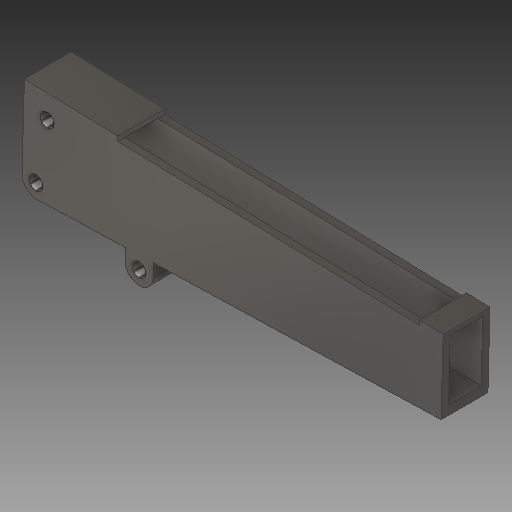
# Autodesk Inventor part: DipperParent
Saved by Autodesk Inventor 2019 (Build 230136000, 136)
## iProperties
Created: 2018-12-27
Part Number: DipperParent
Material: 钢，高强度，低合金
Document SubType Name: Modeling
Designer: JianQiao Hu
Density: 7.85 g/cm^3
Appearance: 钢 - 抛光
Author: JianQiao Hu
Autodesk Inventor part; units mm, degrees
ref_plane "YZ Plane" through (0, 0, 0) normal (1, 0, 0) x (0, 1, 0)
ref_plane "XZ Plane" through (0, 0, 0) normal (0, 1, 0) x (-1, 0, 0)
ref_plane "XY Plane" through (0, 0, 0) normal (0, 0, 1) x (1, 0, 0)
sketch "草图1" plane through (0, 0, 0) normal (0, 0, 1) x (1, 0, 0)
  line L0 (598.9577, 75) -> (600, -74.9964)
  line L1 (-601.0423, 75.1267) -> (600, -74.9964) construction
  line L2 (598.9577, 75) -> (-593.8092, -74.3553) construction
  line L3 (-300, 0) -> (-300, 100)
  line L4 (-300, -100) -> (600, -74.9964)
  line L5 (-300, 100) -> (598.9577, 75)
  line L6 (-300, 0) -> (-300, -100)
  line L7 (599.4789, 0) -> (-300, 0)
  line L8 (0, 0) -> (0, -189.9048)
  dimension "d0" = 150
  dimension "d31" = 75
  dimension "d32" = 0
  dimension "d33" = 100
  dimension "d34" = 100
  dimension "d35" = 100
  dimension "d51" = 300
  constraints: 18 end point, 5 point on line, 3 vertical, 1 perpendicular
  measures "d0" distance of L0.start L0.end
  measures "d31" distance from line of L0.start L7
  measures "d32" distance from line of L8.start L7
  measures "d33" distance from line of L3.end L7
  measures "d34" distance of L3.start L3.end
  measures "d35" distance of L3.start L4.start
  measures "d51" distance between parallel lines of L8 L6
extrude "拉伸1" add sketch "草图1" along normal mid plane 100
sketch "草图2" plane through (0, 0, 0) normal (0, 0, 1) x (1, 0, 0)
  circle A0 centre (-50, -120) radius 15
  line L0 (0, 0) -> (0, -405.8359)
  line L1 (0, 0) -> (-641.787, 0)
  line L2 (-80, -120) -> (-80, -93.888)
  line L3 (-300, -100) -> (600, -74.9964) projected
  line L4 (-20, -92.2211) -> (-20, -120)
  arc A1 (-80, -120) -> (-20, -120) centre (-50, -120) ccw
  dimension "d8" = 30
  dimension "d9" = 120
  dimension "d10" = 50
  dimension "d28" = 30
  constraints: 8 end point, 2 centre point, 2 point on circle, 2 point on line, 2 vertical, 1 coincident, 1 horizontal, 1 tangent
  measures "d8" diameter of A0
  measures "d9" distance from line of L1 A0.centre
  measures "d10" distance from line of L0 A0.centre
  measures "d28" radius of A1
extrude "拉伸2" add sketch "草图2" along normal mid plane 100
fillet "圆角1" radius 30 1 edges at (-300, -100, 0)
sketch "草图4" plane through (0, 0, 50) normal (0, 0, 1) x (1, 0, 0)
  arc A0 (-300, -69.155) -> (-269.1669, -99.1434) centre (-270, -69.155) ccw projected
  circle A1 centre (-270, -69.155) radius 15
  point P0 (0, 0)
  dimension "d15" = 30
  constraints: 1 centre point, 1 coincident
  measures "d15" diameter of A1
extrude "拉伸3" cut sketch "草图4" against normal blind 100
sketch "草图5" plane through (0, 0, 50) normal (0, 0, 1) x (1, 0, 0)
  arc A0 (-300, -69.155) -> (-269.1669, -99.1434) centre (-270, -69.155) ccw projected
  line L0 (-300, -69.155) -> (-300, 100)
  line L1 (598.9577, 75) -> (-300, 100) projected
  line L2 (-300, 100) -> (-300, -69.155) projected
  line L3 (-300, 100) -> (-300, 100)
  line L4 (-300, -69.155) -> (-295.2994, 99.8693)
  line L5 (-295.2994, 99.8693) -> (-300, 100)
  line L6 (598.9577, 75) -> (594.7823, -75.1413)
  line L7 (600, -74.9964) -> (-269.1669, -99.1434) projected
  line L8 (598.9577, 75) -> (600, -74.9964) projected
  line L9 (600, -74.9964) -> (598.9577, 75)
  point P0 (0, 0)
  point P1 (-603.2218, 0)
  point P2 (599.4789, 0)
  dimension "d20" = 90
  constraints: 12 end point, 3 point on line, 1 collinear, 1 horizontal, 1 parallel, 1 other
  measures "d20" angle of L1 L4
extrude "拉伸4" cut sketch "草图5" against normal blind 100 contours L0 L1 L4 | L6 L8 L7
sketch "草图6" plane through (594.7823, -75.1413, 50) normal (0.9996135, -0.0277992, 0) x (0, 0, -1)
  line L0 (0, 0) -> (0, 150.1994) projected
  line L1 (0, 150.1994) -> (100, 150.1994) projected
  line L2 (50, 150.1994) -> (50, 0)
  line L3 (100, 0) -> (0, 0) projected
  line L4 (100, 150.1994) -> (100, 0) projected
  line L5 (15, 151) -> (85, 151)
  line L6 (85, 151) -> (85, 20)
  line L7 (85, 20) -> (15, 20)
  line L8 (15, 20) -> (15, 151)
  line L9 (15, 151) -> (85, 20) construction
  line L10 (85, 151) -> (15, 20) construction
  point P0 (50, 58.5778)
  point P1 (50, 85.5)
  point P2 (0, 100.4456)
  point P3 (0, 175.4618)
  point P4 (100, 175.4618)
  point P5 (100, 100.4456)
  dimension "d21" = 70
  dimension "d22" = 131
  dimension "d63" = 20
  constraints: 14 end point, 3 midpoint, 2 parallel, 1 horizontal, 1 perpendicular, 2 other
  measures "d21" distance of L5.start L5.end
  measures "d22" distance of L5.end L6.end
  measures "d63" distance between parallel lines of L3 L7
extrude "拉伸5" cut sketch "草图6" against normal through all contours L8 L5 L6 L1 | L1 L2 L7 L8 | L2 L1 L6 L7
sketch "草图7" plane through (0, 0, 0) normal (0, 0, 1) x (1, 0, 0)
  arc A0 (-300, -69.155) -> (-269.1669, -99.1434) centre (-270, -69.155) ccw projected
  circle A1 centre (-270, -69.155) radius 42.5
  point P0 (0, 0)
  dimension "d25" = 85
  constraints: 1 centre point, 1 coincident
  measures "d25" diameter of A1
extrude "拉伸6" cut sketch "草图7" along normal mid plane 35
sketch "草图8" plane through (0, 0, 0) normal (0, 0, 1) x (1, 0, 0)
  line L0 (-632.149, 69.2216) -> (221.7891, 45.4736)
  line L1 (-295.2994, 99.8693) -> (-298.9189, -30.2798) projected
  line L2 (598.9577, 75) -> (-295.2994, 99.8693) projected
  circle A0 centre (-246.4307, 58.4948) radius 15
  arc A1 (-276.4191, 59.3288) -> (-216.4423, 57.6608) centre (-246.4307, 58.4948) ccw
  line L3 (-276.4191, 59.3288) -> (-275.3072, 99.3133)
  line L4 (-275.3072, 99.3133) -> (-520.3529, 106.128)
  line L5 (-275.3127, 99.114) -> (-215.3359, 97.446)
  line L6 (598.9522, 74.8007) -> (-295.305, 99.67) projected
  line L7 (-215.3359, 97.446) -> (-216.4423, 57.6608)
  point P0 (0, 0)
  dimension "d36" = 40
  dimension "d37" = 30
  dimension "d38" = 60
  dimension "d39" = 50
  dimension "d40" = 90
  dimension "d41" = 60
  constraints: 10 end point, 7 point on line, 3 perpendicular, 2 centre point, 2 point on circle, 1 coincident, 1 tangent
  measures "d36" distance between parallel lines of L2 L0
  measures "d37" diameter of A0
  measures "d38" diameter of A1
  measures "d39" distance from line of L1 A0.centre
  measures "d40" angle of L2 L3
  measures "d41" distance of L5.start L5.end
extrude "拉伸7" add sketch "草图8" along normal mid plane 70 contours L3 L5 L7 L0 A0 | L0 A0 A1 | A0 L0 | L0 A0
sketch "草图9" plane through (0, 0, 50) normal (0, 0, 1) x (1, 0, 0)
  arc A0 (-276.4191, 59.3288) -> (-216.4423, 57.6608) centre (-246.4307, 58.4948) ccw projected
  circle A1 centre (-246.4307, 58.4948) radius 15
  point P0 (0, 0)
  dimension "d44" = 30
  constraints: 1 centre point, 1 coincident
  measures "d44" diameter of A1
extrude "拉伸8" cut sketch "草图9" against normal through all
sketch "草图10" plane through (-276.4191, 59.3288, -35) normal (-0.9996135, 0.0277992, 0) x (0, 0, 1)
  line L0 (0, 39.8006) -> (70, 39.8006) projected
  line L1 (35, 39.8006) -> (35, -30)
  line L2 (0, -30) -> (70, -30) projected
  line L3 (17.5, 39.8006) -> (52.5, 39.8006)
  line L4 (52.5, 39.8006) -> (52.5, -30)
  line L5 (52.5, -30) -> (17.5, -30)
  line L6 (17.5, -30) -> (17.5, 39.8006)
  line L7 (17.5, 39.8006) -> (52.5, -30) construction
  line L8 (52.5, 39.8006) -> (17.5, -30) construction
  point P0 (35, -51.6216)
  point P1 (35, 4.9003)
  dimension "d47" = 35
  constraints: 14 end point, 5 midpoint, 2 parallel, 1 horizontal, 1 perpendicular, 1 point on line
  measures "d47" distance between parallel lines of L4 L6
extrude "拉伸9" cut sketch "草图10" against normal blind 60
sketch "草图13" plane through (-295.2994, 99.8693, 50) normal (0.0277992, 0.9996135, 0) x (0.9996135, -0.0277992, 0)
  line L0 (0, 15) -> (0, 85) projected
  line L1 (0, 50) -> (323.6348, 50)
  line L2 (0, 100) -> (31.6549, 100) projected
  line L3 (200, 0) -> (0, 0)
  line L4 (0, 0) -> (0, 100)
  line L5 (0, 100) -> (200, 100)
  line L6 (200, 100) -> (200, 0)
  line L7 (200, 0) -> (0, 100) construction
  line L8 (0, 0) -> (200, 100) construction
  line L9 (894.6029, 100) -> (894.6029, 0) projected
  line L10 (844.6029, 100) -> (894.6029, 100)
  line L11 (894.6029, 100) -> (894.6029, 0)
  line L12 (894.6029, 0) -> (844.6029, 0)
  line L13 (844.6029, 0) -> (844.6029, 100)
  line L14 (844.6029, 100) -> (894.6029, 0) construction
  line L15 (894.6029, 100) -> (844.6029, 0) construction
  point P0 (297.9616, 50)
  point P1 (100, 50)
  point P2 (869.6029, 50)
  dimension "d64" = 200
  dimension "d65" = 50
  constraints: 26 end point, 5 midpoint, 4 parallel, 3 horizontal, 2 perpendicular, 1 point on line
  measures "d64" distance of L2.start L5.end
  measures "d65" distance of L10.start L10.end
extrude "拉伸12" add sketch "草图13" along normal blind 10
